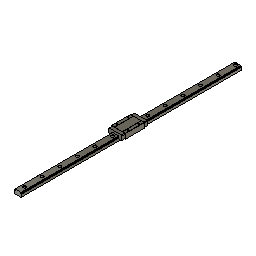
MGN15 rail 500mm, X travel 350+20mm v1 (Autodesk Fusion 360 design; units mm, degrees)
Autodesk Fusion 360 part; units mm, degrees
sketch "Sketch1" plane through (0, 0, 0) normal (0, 1, 0) x (1, 0, 0) in component "Rail, 500mm"
  line L0 (16.183, -28.3382) -> (31.183, -28.3382)
  line L1 (31.183, -18.3382) -> (16.183, -18.3382)
  line L2 (11.1951, -25.8382) -> (35.1106, -25.8382) construction
  line L3 (23.683, -28.3382) -> (23.683, -18.3382) construction
  line L4 (17.1512, -25.8382) -> (17.1512, -26.0882)
  line L5 (17.1512, -26.0882) -> (16.9012, -26.0882)
  arc A0 (16.183, -26.8065) -> (16.9012, -26.0882) centre (15.933, -25.8382) ccw
  arc A1 (16.9012, -25.5882) -> (16.183, -24.87) centre (15.933, -25.8382) ccw
  line L6 (17.1512, -25.5882) -> (16.9012, -25.5882)
  line L7 (17.1512, -25.8382) -> (17.1512, -25.5882)
  arc A2 (30.4647, -26.0882) -> (31.183, -26.8065) centre (31.433, -25.8382) ccw
  line L8 (30.2147, -26.0882) -> (30.4647, -26.0882)
  line L9 (30.2147, -25.8382) -> (30.2147, -26.0882)
  line L10 (30.2147, -25.8382) -> (30.2147, -25.5882)
  line L11 (30.2147, -25.5882) -> (30.4647, -25.5882)
  arc A3 (31.183, -24.87) -> (30.4647, -25.5882) centre (31.433, -25.8382) ccw
  line L12 (16.183, -18.3382) -> (16.183, -24.87)
  line L13 (16.183, -26.8065) -> (16.183, -28.3382)
  line L14 (31.183, -28.3382) -> (31.183, -26.8065)
  line L15 (31.183, -24.87) -> (31.183, -18.3382)
  dimension "d1" = 15
  dimension "d2" = 10
  dimension "d3" = 2.5
  dimension "d4" = 0.25
  dimension "d5" = 0.25
  dimension "d6" = 1
  dimension "d7" = 0.25
  dimension "d65" = 0
  dimension "d66" = 0
  dimension "d67" = 0
  dimension "d68" = 0
  dimension "d75" = 0
  dimension "d76" = 0
  dimension "d77" = 0
  dimension "d78" = 0
  constraint horizontal L0
  constraint vertical L14
  constraint horizontal L1
  constraint vertical L12
  constraint perpendicular L2 L14
  constraint midpoint L0 L3.start
  constraint midpoint L1 L3.end
  constraint coincident L2 L4.start
  constraint perpendicular L2 L4
  constraint perpendicular L4 L5
  constraint coincident A0.start L12
  constraint coincident L2 A0.centre
  constraint symmetric L2 L4.start L7.start
  constraint symmetric L2 L4.end L6.start
  constraint symmetric L2 L5.end A1.start
  constraint symmetric L2 A0.start A1.end
  constraint symmetric L2 A0 A1
  constraint symmetric L3 L4.start L9.start
  constraint symmetric L3 L4.end L8.start
  constraint symmetric L3 L5.end A2.start
  constraint symmetric L3 A0.start A2.end
  constraint symmetric L3 A0 A2
  constraint symmetric L3 A1.end A3.start
  constraint symmetric L3 A1.start L11.end
  constraint symmetric L3 A1 A3
  constraint symmetric L3 L6.start L10.end
  constraint collinear L12 L13
  constraint collinear L14 L15
  measures "d1" distance of L0.start L0.end
  measures "d2" distance of L0.start L1.end
  measures "d3" distance of L0 L2
  measures "d4" distance of L2 L5
  measures "d5" distance of A0.centre L12
  measures "d6" radius of A0
  measures "d7" distance of L4 L5.end
extrude "Extrude1" add sketch "Sketch1" along normal blind 500 makes body 1 in component "Rail, 500mm"
chamfer "Chamfer1" distance 0.75 angle 45 4 edges at (31.183, 250, 28.3382) (31.183, 250, 18.3382) (16.183, 250, 28.3382) (16.183, 250, 18.3382) on bodies 1 in component "Rail, 500mm"
sketch "Sketch2" plane through (0, 0, 28.3382) normal (0, 0, 1) x (-1, 0, 0) in component "Rail, 500mm"
  line L0 (-16.933, -500) -> (-16.933, 0)
  line L1 (-16.933, 0) -> (-30.433, 0)
  line L2 (-30.433, 0) -> (-30.433, -500)
  line L3 (-30.433, -500) -> (-16.933, -500)
  circle A0 centre (-23.683, -15) radius 3
  line L4 (-31.183, 0) -> (-16.183, 0)
  circle A1 centre (-23.683, -15) radius 1.75
  point P0 (-23.683, 0)
  dimension "d11" = 15
  dimension "d12" = 6
  dimension "d13" = 3.5
  constraint concentric A0 A1
  constraint midpoint L4 P0
  constraint vertical A0.centre P0
  measures "d11" distance of A0.centre L4
  measures "d12" diameter of A0
  measures "d13" diameter of A1
extrude "Extrude2" cut sketch "Sketch2" against normal blind 10 contours A1 bodies 1 in component "Rail, 500mm"
extrude "Extrude3" cut sketch "Sketch2" against normal blind 4.5 contours A0 bodies 1 in component "Rail, 500mm"
chamfer "Chamfer2" distance 0.5 angle 45 2 edges at (25.3146, 15.6328, 18.3382) (26.48, 13.9152, 28.3382) on bodies 1 in component "Rail, 500mm"
pattern_linear "R-Pattern1" count 112 spacing 40 along (0, 1, 0) of 5 faces at (20.3538, 15.1662, 28.1716) (20.6979, 15.2987, 26.5049) (21.1108, 15.149, 23.8382) (21.9417, 15.1742, 22.1716) (22.1558, 16.417, 18.5049) on bodies 1 in component "Rail, 500mm"
sketch "Sketch1 (2)" plane through (0, 0, 0) normal (0, 1, 0) x (1, 0, 0) in component "sliding block"
  line L0 (23.683, -28.3382) -> (23.683, -18.3382) construction
  line L1 (11.1951, -25.8382) -> (35.1106, -25.8382) construction
  line L2 (15.683, -22.3382) -> (7.683, -22.3382)
  line L3 (7.683, -22.3382) -> (7.683, -34.3382)
  line L4 (7.683, -34.3382) -> (39.683, -34.3382)
  line L5 (39.683, -34.3382) -> (39.683, -22.3382)
  line L6 (39.683, -22.3382) -> (31.683, -22.3382)
  line L7 (31.683, -22.3382) -> (31.683, -28.8382)
  line L8 (31.683, -28.8382) -> (15.683, -28.8382)
  line L9 (15.683, -28.8382) -> (15.683, -22.3382)
  line L10 (16.183, -28.3382) -> (31.183, -28.3382)
  line L11 (16.183, -18.3382) -> (16.183, -24.87)
  line L12 (31.183, -24.87) -> (31.183, -18.3382)
  line L13 (31.183, -18.3382) -> (16.183, -18.3382)
  dimension "d23" = 32
  dimension "d24" = 16
  dimension "d25" = 12
  dimension "d26" = 16
  dimension "d27" = 0.5
  dimension "d28" = 0.5
  constraint parallel L1 L2
  constraint perpendicular L1 L3
  constraint perpendicular L3 L4
  constraint perpendicular L4 L5
  constraint perpendicular L5 L6
  constraint perpendicular L1 L7
  constraint perpendicular L5 L8
  constraint perpendicular L2 L9
  constraint collinear L2 L6
  constraint equal L2 L6
  measures "d23" distance of L3 L5
  measures "d24" distance of L0 L5
  measures "d25" distance of L4 L6
  measures "d26" distance of L4 L13
  measures "d27" distance of L9 L11
  measures "d28" distance of L8 L10
extrude "Extrude1'" add sketch "Sketch1 (2)" along normal blind 43.4 separate body makes body 2 in component "sliding block"
sketch "Sketch2 (2)" plane through (0, 0, 0) normal (0, 1, 0) x (1, 0, 0) in component "sliding block"
  line L0 (8.433, -22.3382) -> (8.433, -33.5882)
  line L1 (8.433, -33.5882) -> (38.933, -33.5882)
  line L2 (38.933, -33.5882) -> (38.933, -22.3382)
  line L3 (15.683, -22.3382) -> (15.683, -28.8382)
  line L4 (15.683, -28.8382) -> (31.683, -28.8382)
  line L5 (31.683, -28.8382) -> (31.683, -22.3382)
  line L6 (31.683, -22.3382) -> (39.683, -22.3382)
  line L7 (39.683, -22.3382) -> (39.683, -34.3382)
  line L8 (39.683, -34.3382) -> (7.683, -34.3382)
  line L9 (7.683, -34.3382) -> (7.683, -22.3382)
  line L10 (7.683, -22.3382) -> (15.683, -22.3382)
  dimension "d31" = 0.75
  dimension "d32" = 0.75
  dimension "d33" = 0.75
  constraint vertical L0
  constraint perpendicular L0 L1
  constraint perpendicular L1 L2
  constraint coincident L10 L0.start
  constraint coincident L6 L2.end
  measures "d31" distance of L0 L9
  measures "d32" distance of L1 L8
  measures "d33" distance of L2 L7
extrude "Extrude2'" add sketch "Sketch2 (2)" along normal blind 50.65 and the other way blind 7.35 contours L0 L1 L2 L3 L4 L5 L6 L10 bodies 2 in component "sliding block"
sketch "Sketch3" plane through (0, 0, 34.3382) normal (0, 0, 1) x (-1, 0, 0) in component "sliding block"
  line L0 (-7.683, 0) -> (-39.683, 0)
  line L1 (-39.683, 0) -> (-39.683, -43.4)
  line L2 (-39.683, -43.4) -> (-7.683, -43.4)
  line L3 (-7.683, -43.4) -> (-7.683, 0)
  circle A0 centre (-11.183, -9.2) radius 1.5
  circle A1 centre (-36.183, -9.2) radius 1.5
  circle A2 centre (-11.183, -34.2) radius 1.5
  circle A3 centre (-36.183, -34.2) radius 1.5
  line L4 (-14.683, -43.4) -> (-14.683, 0)
  line L5 (-32.683, -43.4) -> (-32.683, 0)
  dimension "d38" = 3.5
  dimension "d39" = 9.2
  dimension "d42" = -25
  dimension "d43" = -25
  dimension "d44" = 3
  dimension "d49" = 7
  dimension "d50" = 7
  constraint coincident L2 L4.start
  constraint perpendicular L2 L4
  constraint coincident L0 L4.end
  constraint coincident L2 L5.start
  constraint perpendicular L2 L5
  constraint coincident L0 L5.end
  measures "d38" distance of L3 A0.centre
  measures "d39" distance of L0 A0.centre
  measures "d44" diameter of A0
  measures "d49" distance of L3 L4
  measures "d50" distance of L1 L5
extrude "Extrude3'" cut sketch "Sketch3" against normal blind 8 contours A0 | A1 | A2 | A3 bodies 2 in component "sliding block"
extrude "Extrude5" cut sketch "Sketch3" against normal blind 0.5 contours L0 L2 L4 L5 bodies 2 in component "sliding block"
chamfer "Chamfer3" distance 0.5 angle 45 12 edges at (11.183, 0, 34.3382) (39.683, 0, 28.3382) (36.183, 0, 34.3382) (39.683, 43.4, 28.3382) (36.183, 43.4, 34.3382) (11.183, 43.4, 34.3382) (7.683, 21.7, 34.3382) (39.683, 21.7, 34.3382) (39.683, 21.7, 22.3382) (7.683, 21.7, 22.3382) (7.683, 0, 28.3382) (7.683, 43.4, 28.3382) on bodies 2 in component "sliding block"
chamfer "Chamfer4" distance 1.25 angle 45 8 edges at (38.933, -3.675, 33.5882) (8.433, -3.675, 33.5882) (38.933, -3.675, 22.3382) (38.933, 47.025, 22.3382) (38.933, 47.025, 33.5882) (8.433, 47.025, 33.5882) (8.433, 47.025, 22.3382) (8.433, -3.675, 22.3382) on bodies 2 in component "sliding block"
component "MGN15H Linear rail, 500mm" placed x (1, 0, 0) y (0, 1, 0) z (0, 0, 1) at (0, 0, 0)
component "sliding block" placed x (1, 0, 0) y (0, 1, 0) z (0, 0, 1) at (0, 228.35, 0.75)
component "Rail, 500mm" placed x (1, 0, 0) y (0, 1, 0) z (0, 0, 1) at (0, 0, 0) in component "MGN15H Linear rail, 500mm"
equation "d5 = d6 / 4"
equation "d24 = d23 / 2"
equation "d28 = d27"
equation "d32 = d31"
equation "d33 = d31"
equation "d34 = 58 mm - ( ( 58 - 43.3 ) / 2 ) * 1 mm"
equation "d36 = ( ( 58 - 43.3 ) / 2 ) * 1 mm"
equation "d39 = ( ( 43.4 - 25 ) / 2 ) * 1 mm"
equation "d50 = d49"
equation "d73 = ( -Total_travel / 2 mm ) * 1 mm"
equation "d74 = Total_travel / 2"
equation "Total_travel = Max_Part_size + Extra_travle_rspace"
equation "Max_Part_size = 350 mm"
equation "Extra_travle_rspace = 20 mm"
